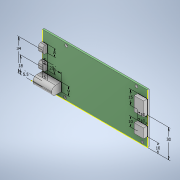
# Autodesk Inventor part: EVAL_ADICUP360
Saved by Autodesk Inventor 2021 (Build 250183000, 183)
## iProperties
Created: 2019-11-04
Part Number: EVAL_ADICUP360
Material: Generic
Document SubType Name: Modeling
Designer: jgray
Density: 1 g/cm^3
Appearance: Default
Author: jgray
Autodesk Inventor part; units mm, degrees
ref_plane "YZ Plane" through (0, 0, 0) normal (1, 0, 0) x (0, 1, 0)
ref_plane "XZ Plane" through (0, 0, 0) normal (0, 1, 0) x (-1, 0, 0)
ref_plane "XY Plane" through (0, 0, 0) normal (0, 0, 1) x (1, 0, 0)
sketch "Sketch1" plane through (0, 0, 0) normal (0, 0, 1) x (1, 0, 0)
  line L0 (11.35, 0) -> (123.35, 0)
  line L1 (123.35, 0) -> (123.35, 53.25)
  line L2 (123.35, 53.25) -> (11.35, 53.25)
  line L3 (11.35, 53.25) -> (11.35, 0)
  line L4 (13.2018, 50.8) -> (120.6255, 50.8) construction
  line L5 (12.1008, 2.54) -> (119.6818, 2.54) construction
  point P0 (0, 0)
  point P1 (0, 0)
  point P2 (36.84, 50.8)
  point P3 (111.77, 50.8)
  point P4 (118.12, 2.54)
  point P5 (35.57, 2.54)
  dimension "d0" = 112
  dimension "d1" = 53.25
  dimension "d2" = 48.26
  dimension "d3" = 2.45
  dimension "d4" = 74.93
  dimension "d5" = 82.55
  dimension "d6" = 6.35
  dimension "d7" = 5.23
  dimension "d38" = 100.42
  dimension "d39" = 1.27
  constraints: 12 end point, 4 point on line, 3 horizontal, 2 parallel, 1 perpendicular
  measures "d0" distance of L2.end L1.end
  measures "d1" distance of L1.end L0.end
  measures "d2" distance between parallel lines of L5 L4
  measures "d3" distance between parallel lines of L2 L4
  measures "d4" distance of point (111.77, 50.8) point (36.84, 50.8)
  measures "d5" distance of point (118.12, 2.54) point (35.57, 2.54)
  measures "d6" horizontal distance of point (118.12, 2.54) point (111.77, 50.8)
  measures "d7" distance from line of L1 point (118.12, 2.54)
  measures "d38" distance from line of L3 point (111.77, 50.8)
  measures "d39" horizontal distance of point (35.57, 2.54) point (36.84, 50.8)
extrude "Extrusion1" add sketch "Sketch1" along normal blind 1.8
hole "Hole1" at (36.84, 50.8, 0) at (111.77, 50.8, 0) at (118.12, 2.54, 0) at (35.57, 2.54, 0) direction (0, 0, 1) diameter 3.1 end through all
sketch "Sketch2" plane through (0, 0, 1.8) normal (0, 0, 1) x (1, 0, 0)
  line L0 (123.35, 0) -> (123.35, 53.25) projected
  line L1 (123.35, 10) -> (113.35, 10)
  line L2 (113.35, 10) -> (113.35, 20)
  line L3 (113.35, 20) -> (123.35, 20)
  line L4 (123.35, 20) -> (123.35, 10)
  line L5 (11.35, 0) -> (123.35, 0) projected
  line L6 (123.35, 45) -> (113.35, 45)
  line L7 (113.35, 45) -> (113.35, 30)
  line L8 (113.35, 30) -> (123.35, 30)
  line L9 (123.35, 30) -> (123.35, 45)
  line L10 (11.35, 53.25) -> (11.35, 0) projected
  line L11 (11.35, 5.5) -> (31.35, 5.5)
  line L12 (31.35, 5.5) -> (31.35, 14.5)
  line L13 (31.35, 14.5) -> (11.35, 14.5)
  line L14 (11.35, 14.5) -> (11.35, 5.5)
  line L15 (11.35, 42) -> (16.35, 42)
  line L16 (16.35, 42) -> (16.35, 34)
  line L17 (16.35, 34) -> (11.35, 34)
  line L18 (11.35, 34) -> (11.35, 42)
  line L19 (11.35, 26) -> (16.35, 26)
  line L20 (16.35, 26) -> (16.35, 18)
  line L21 (16.35, 18) -> (11.35, 18)
  line L22 (11.35, 18) -> (11.35, 26)
  point P0 (0, 0)
  dimension "d17" = 10
  dimension "d18" = 10
  dimension "d19" = 10
  dimension "d20" = 10
  dimension "d21" = 15
  dimension "d22" = 30
  dimension "d23" = 20
  dimension "d24" = 9
  dimension "d25" = 5
  dimension "d26" = 8
  dimension "d27" = 5
  dimension "d28" = 8
  dimension "d29" = 5.5
  dimension "d30" = 18
  dimension "d31" = 34
  constraints: 40 end point, 10 parallel, 5 horizontal, 5 perpendicular, 5 point on line
  measures "d17" distance of L2.end L3.end
  measures "d18" distance of L1.end L2.end
  measures "d19" distance between parallel lines of L5 L1
  measures "d20" distance of L8.end L7.end
  measures "d21" distance of L7.end L6.end
  measures "d22" distance between parallel lines of L8 L5
  measures "d23" distance of L13.end L12.end
  measures "d24" distance of L12.end L11.end
  measures "d25" distance of L16.end L17.end
  measures "d26" distance of L15.end L16.end
  measures "d27" distance of L20.end L21.end
  measures "d28" distance of L19.end L20.end
  measures "d29" distance between parallel lines of L5 L11
  measures "d30" distance between parallel lines of L21 L5
  measures "d31" distance between parallel lines of L17 L5
extrude "Extrusion2" add sketch "Sketch2" along normal blind 4
extrude "Extrusion3" add sketch "Sketch2" along normal blind 10 contours L10 L13 L12 L11
fillet "Fillet1" radius 4 2 edges at (21.35, 14.5, 11.8) (21.35, 5.5, 11.8)
fillet "Fillet2" radius 2 4 edges at (13.85, 26, 5.8) (13.85, 18, 5.8) (13.85, 34, 5.8) (13.85, 42, 5.8)
body "Solid1"
